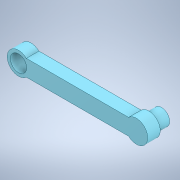
# Autodesk Inventor part: Component39
Saved by Autodesk Inventor 2022 (Build 260153000, 153)
## iProperties
Created: 2022-01-29
Part Number: Component39
Material: Generic
Document SubType Name: Modeling
Designer: Administrator
Density: 1 g/cm^3
Appearance: Default
width: 6,500 mm
d6: 35,000 mm
thickness: 5,000 mm
R: 6,500 mm
R1: 9,000 mm
Title: Component39
Author: Administrator
Autodesk Inventor part; units mm, degrees
ref_plane "YZ Plane" through (0, 0, 0) normal (1, 0, 0) x (0, 1, 0)
ref_plane "XZ Plane" through (0, 0, 0) normal (0, 1, 0) x (-1, 0, 0)
ref_plane "XY Plane" through (0, 0, 0) normal (0, 0, 1) x (1, 0, 0)
sketch "Sketch2" plane through (0, 0, 0) normal (0, 0, 1) x (1, 0, 0)
  circle A0 centre (-26.3625, 10.7058) radius 3.25
  circle A1 centre (20.6375, 10.7058) radius 3.25
  arc A2 (17.525, 7.4558) -> (17.525, 13.9558) centre (20.6375, 10.7058) ccw
  line L0 (17.525, 13.9558) -> (-23.25, 13.9558)
  arc A3 (-23.25, 13.9558) -> (-23.25, 7.4558) centre (-26.3625, 10.7058) ccw
  line L1 (-33.5959, 10.7058) -> (33.9179, 10.7058) construction
  line L2 (17.525, 7.4558) -> (-23.25, 7.4558)
  dimension "d4" = 47
  dimension "d8" = 6.5
  dimension "d10" = 9
  dimension "d11" = 6.5
  constraints: 6 end point, 4 centre point, 4 point on circle, 2 coincident, 2 equal radius, 2 point on line, 2 symmetric about line, 1 horizontal, 1 parallel
  measures "d4" distance of A1.centre A0.centre
  measures "d8" diameter of A0
  measures "d10" diameter of A3
  measures "d11" distance between parallel lines of L2 L0
extrude "Extrusion1" add sketch "Sketch2" along normal blind 5 contours A1 | L2 A3 L0 A2
extrude "Extrusion2" add sketch "Sketch2" against normal blind 5 contours A1
equation "\"d8\" = R"
equation "\"d10\" = R1"
equation "\"d11\" = width"
equation "\"d0\" = thickness"
equation "\"d2\" = thickness"
equation "\"R\" = 6.5"
equation "\"thickness\" = 5"
equation "\"d6\" = 35"
equation "\"width\" = 6.5"
equation "\"R1\" = 9"
body "Solid1"
